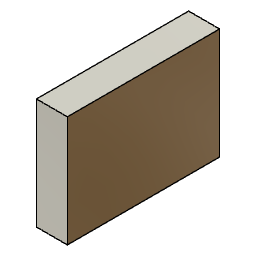
control_panel_support_right (Autodesk Fusion 360 design; units mm, degrees)
Autodesk Fusion 360 part; units mm, degrees
sketch "Control Panel Support" plane through (0, 0, 0) normal (1, 0, 0) x (0, 1, 0)
  line L0 (0, 0) -> (59, 0)
  line L1 (59, 0) -> (59, 43)
  line L2 (59, 43) -> (0, 43)
  line L3 (0, 43) -> (0, 0)
  dimension "d1" = 59
  dimension "d2" = 43
  constraint horizontal L0
  constraint vertical L1
  constraint horizontal L2
  constraint vertical L3
  constraint coincident L0.start L3.end
  measures "d1" distance of L0.start L0.end
  measures "d2" distance of L0.end L1.end
extrude "Extrude1" add sketch "Control Panel Support" along normal blind 12
equation "d1 = 65 mm - mdfThickness"
equation "pineThickness = 12 mm" comment "Thickness of the pine planks"
equation "d4 = pineThickness"
equation "mdfThickness = 6 mm" comment "Thickness of the MDF board"
named bodies: "Control Panel Support Right"
